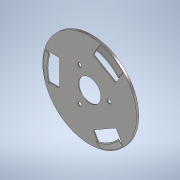
# Autodesk Inventor part: Tarcza_OsłonaB
Saved by Autodesk Inventor 2022 (Build 260153000, 153)
## iProperties
Created: 2021-06-26
Part Number: Tarcza_OsłonaB
Material: Stal, galwanizowana
Document SubType Name: Modeling
Designer: Matik
Density: 7.85 g/cm^3
Appearance: Galwanizowana
Author: Matik
Autodesk Inventor part; units mm, degrees
ref_plane "YZ Plane" through (0, 0, 0) normal (1, 0, 0) x (0, 1, 0)
ref_plane "Płaszczyzna konstrukcyjna1" through (2.025, 0, 2) normal (0, 0, 1) x (-1, 0, 0)
sketch "Szkic1" plane through (2.025, 0, 2) normal (0, 0, 1) x (-1, 0, 0)
  line L0 (22.5, 22.5) -> (22.5, 27.5) projected
  line L1 (22.5, 27.5) -> (27.5, 27.5) projected
  line L2 (27.5, 27.5) -> (27.5, 22.5) projected
  line L3 (27.5, 22.5) -> (22.5, 22.5) projected
  line L4 (-22.5, 27.5) -> (-22.5, 22.5) projected
  line L5 (-22.5, 22.5) -> (-27.5, 22.5) projected
  line L6 (-27.5, 22.5) -> (-27.5, 27.5) projected
  line L7 (-27.5, 27.5) -> (-22.5, 27.5) projected
  line L8 (22.5, -22.5) -> (27.5, -22.5) projected
  line L9 (27.5, -22.5) -> (27.5, -27.5) projected
  line L10 (27.5, -27.5) -> (22.5, -27.5) projected
  line L11 (22.5, -27.5) -> (22.5, -22.5) projected
  line L12 (-27.5, -27.5) -> (-27.5, -22.5) projected
  line L13 (-27.5, -22.5) -> (-22.5, -22.5) projected
  line L14 (-22.5, -22.5) -> (-22.5, -27.5) projected
  line L15 (-22.5, -27.5) -> (-27.5, -27.5) projected
  arc A0 (-56.2827, -21.6239) -> (-57.5723, -24.3244) centre (-55.73, -23.5461) ccw projected
  arc A1 (-57.5723, -24.3244) -> (7.7206, -62.0213) centre (0, 0) ccw projected
  arc A2 (7.7206, -62.0213) -> (9.4144, -59.5542) centre (7.4735, -60.0366) ccw projected
  arc A3 (46.8682, -37.9302) -> (9.4144, -59.5542) centre (31.25, -54.1266) ccw projected
  arc A4 (46.8682, -37.9302) -> (49.8517, -37.6969) centre (48.2565, -36.4906) ccw projected
  arc A5 (49.8517, -37.6969) -> (49.8517, 37.6969) centre (0, 0) ccw projected
  arc A6 (49.8517, 37.6969) -> (46.8682, 37.9302) centre (48.2565, 36.4906) ccw projected
  arc A7 (9.4144, 59.5542) -> (46.8682, 37.9302) centre (31.25, 54.1266) ccw projected
  arc A8 (9.4144, 59.5542) -> (7.7206, 62.0213) centre (7.4735, 60.0366) ccw projected
  arc A9 (7.7206, 62.0213) -> (-57.5723, 24.3244) centre (0, 0) ccw projected
  arc A10 (-57.5723, 24.3244) -> (-56.2827, 21.6239) centre (-55.73, 23.5461) ccw projected
  arc A11 (-56.2827, -21.6239) -> (-56.2827, 21.6239) centre (-62.5, 0) ccw projected
  line L16 (-6.5766, 42.391) -> (-33.4234, 26.891) projected
  arc A12 (-36.1554, 27.6231) -> (-33.4234, 26.891) centre (-34.4234, 28.6231) ccw projected
  line L17 (-36.1554, 27.6231) -> (-42.0186, 37.7784) projected
  arc A13 (-41.9061, 39.9519) -> (-42.0186, 37.7784) centre (-40.2866, 38.7784) ccw projected
  arc A14 (-13.6463, 56.2677) -> (-41.9061, 39.9519) centre (-9.5156, 16.4816) ccw projected
  arc A15 (-11.7077, 55.2784) -> (-13.6463, 56.2677) centre (-13.4398, 54.2784) ccw projected
  line L18 (-11.7077, 55.2784) -> (-5.8446, 45.1231) projected
  arc A16 (-6.5766, 42.391) -> (-5.8446, 45.1231) centre (-7.5766, 44.1231) ccw projected
  line L19 (-33.4234, -26.891) -> (-6.5766, -42.391) projected
  arc A17 (-5.8446, -45.1231) -> (-6.5766, -42.391) centre (-7.5766, -44.1231) ccw projected
  line L20 (-5.8446, -45.1231) -> (-11.7077, -55.2784) projected
  arc A18 (-13.6463, -56.2677) -> (-11.7077, -55.2784) centre (-13.4398, -54.2784) ccw projected
  arc A19 (-41.9061, -39.9519) -> (-13.6463, -56.2677) centre (-9.5156, -16.4816) ccw projected
  arc A20 (-42.0186, -37.7784) -> (-41.9061, -39.9519) centre (-40.2866, -38.7784) ccw projected
  line L21 (-42.0186, -37.7784) -> (-36.1554, -27.6231) projected
  arc A21 (-33.4234, -26.891) -> (-36.1554, -27.6231) centre (-34.4234, -28.6231) ccw projected
  line L22 (40, -15.5) -> (40, 15.5) projected
  arc A22 (42, 17.5) -> (40, 15.5) centre (42, 15.5) ccw projected
  line L23 (42, 17.5) -> (53.7264, 17.5) projected
  arc A23 (55.5524, 16.3158) -> (53.7264, 17.5) centre (53.7264, 15.5) ccw projected
  arc A24 (55.5524, -16.3158) -> (55.5524, 16.3158) centre (19.0313, 0) ccw projected
  arc A25 (53.7264, -17.5) -> (55.5524, -16.3158) centre (53.7264, -15.5) ccw projected
  line L24 (53.7264, -17.5) -> (42, -17.5) projected
  arc A26 (40, -15.5) -> (42, -17.5) centre (42, -15.5) ccw projected
  arc A27 (-21.36, 10) -> (-19.6163, 11.0204) centre (-21.36, 12) ccw projected
  arc A28 (0.2642, 22.4984) -> (-19.6163, 11.0204) centre (0, 0) ccw projected
  arc A29 (0.2642, 22.4984) -> (2.0198, 23.4983) centre (0.2877, 24.4983) ccw projected
  line L25 (2.0198, 23.4983) -> (2.5897, 24.4856) projected
  arc A30 (19.9103, 14.4856) -> (2.5897, 24.4856) centre (11.25, 19.4856) ccw projected
  line L26 (19.9103, 14.4856) -> (19.3403, 13.4983) projected
  arc A31 (19.3403, 13.4983) -> (19.3521, 11.478) centre (21.0723, 12.4983) ccw projected
  arc A32 (19.3521, -11.478) -> (19.3521, 11.478) centre (0, 0) ccw projected
  arc A33 (19.3521, -11.478) -> (19.3403, -13.4983) centre (21.0723, -12.4983) ccw projected
  line L27 (19.3403, -13.4983) -> (19.9103, -14.4856) projected
  arc A34 (2.5897, -24.4856) -> (19.9103, -14.4856) centre (11.25, -19.4856) ccw projected
  line L28 (2.5897, -24.4856) -> (2.0198, -23.4983) projected
  arc A35 (2.0198, -23.4983) -> (0.2642, -22.4984) centre (0.2877, -24.4983) ccw projected
  arc A36 (-19.6163, -11.0204) -> (0.2642, -22.4984) centre (0, 0) ccw projected
  arc A37 (-19.6163, -11.0204) -> (-21.36, -10) centre (-21.36, -12) ccw projected
  line L29 (-21.36, -10) -> (-22.5, -10) projected
  arc A38 (-22.5, 10) -> (-22.5, -10) centre (-22.5, 0) ccw projected
  line L30 (-22.5, 10) -> (-21.36, 10) projected
  circle A39 centre (0, 0) radius 62.5
  circle A40 centre (-26, 0) radius 2.5 projected
  circle A41 centre (13, -22.5167) radius 2.5 projected
  circle A42 centre (13, 22.5167) radius 2.5 projected
  arc A43 (0.2642, 22.4984) -> (-19.6163, 11.0204) centre (0, 0) ccw projected
  arc A44 (-21.36, 10) -> (-19.6163, 11.0204) centre (-21.36, 12) ccw projected
  line L31 (-21.36, 10) -> (-22.5, 10) projected
  arc A45 (-22.5, 10) -> (-22.5, -10) centre (-22.5, 0) ccw projected
  line L32 (-22.5, -10) -> (-21.36, -10) projected
  arc A46 (-19.6163, -11.0204) -> (-21.36, -10) centre (-21.36, -12) ccw projected
  arc A47 (-19.6163, -11.0204) -> (0.2642, -22.4984) centre (0, 0) ccw projected
  arc A48 (2.0198, -23.4983) -> (0.2642, -22.4984) centre (0.2877, -24.4983) ccw projected
  line L33 (2.0198, -23.4983) -> (2.5897, -24.4856) projected
  arc A49 (2.5897, -24.4856) -> (19.9103, -14.4856) centre (11.25, -19.4856) ccw projected
  line L34 (19.9103, -14.4856) -> (19.3403, -13.4983) projected
  arc A50 (19.3521, -11.478) -> (19.3403, -13.4983) centre (21.0723, -12.4983) ccw projected
  arc A51 (19.3521, -11.478) -> (19.3521, 11.478) centre (0, 0) ccw projected
  arc A52 (19.3403, 13.4983) -> (19.3521, 11.478) centre (21.0723, 12.4983) ccw projected
  line L35 (19.3403, 13.4983) -> (19.9103, 14.4856) projected
  arc A53 (19.9103, 14.4856) -> (2.5897, 24.4856) centre (11.25, 19.4856) ccw projected
  line L36 (2.5897, 24.4856) -> (2.0198, 23.4983) projected
  arc A54 (0.2642, 22.4984) -> (2.0198, 23.4983) centre (0.2877, 24.4983) ccw projected
  circle A55 centre (0, 0) radius 15 projected
  point P0 (2.025, 0)
  point P1 (49.8517, -37.6969)
  point P2 (49.8517, 37.6969)
  point P3 (-57.5723, 24.3244)
  point P4 (7.7206, -62.0213)
  constraints: 1 centre point, 1 coincident, 1 concentric
extrude "Wyciągnięcie proste1" add sketch "Szkic1" along normal blind 1 contours L0 L1 L2 L3 | L4 L5 L6 L7 | L8 L9 L10 L11 | L12 L13 L14 L15 | A11 A10 A9 A8 A7 A6 A5 A4 A3 A2 A1 A0 | A0 A39 A10 A11 | A2 A3 A4 A39 | A39 A6 A7 A8 | A27 A28 A29 L25 A30 L26 A31 A32 A33 L27 A34 L28 A35 A36 A37 L29 A38 L30
sketch "Szkic2" plane through (2.025, 0, 2) normal (0, 0, -1) x (-1, 0, 0)
  circle A0 centre (0, 0) radius 61
  circle A1 centre (0, 0) radius 62.5
  point P0 (2.025, 0)
  dimension "d2" = 122
  dimension "d3" = 125
  constraints: 2 centre point, 1 coincident
  measures "d2" diameter of A0
  measures "d3" diameter of A1
extrude "Wyciągnięcie proste2" add sketch "Szkic2" along normal blind 2
ref_plane "Płaszczyzna konstrukcyjna2" through (2.025, 0, 5) normal (0, 0, 1) x (1, 0, 0)
sketch "Szkic5" plane through (2.025, 0, 5) normal (0, 0, 1) x (1, 0, 0)
  arc A0 (-50.7797, 16.8426) -> (-50.7797, -16.8426) centre (0, 0) ccw
  arc A1 (-52.2558, 17.156) -> (-52.2558, -17.156) centre (0, 0) ccw
  line L0 (-42, -17.5) -> (-53.7264, -17.5) projected
  line L1 (-51.2543, -17.5) -> (-51.7808, -17.5)
  line L2 (-53.7264, 17.5) -> (-42, 17.5) projected
  line L3 (-51.2543, 17.5) -> (-51.7808, 17.5)
  arc A2 (-51.2543, -17.5) -> (-50.7797, -16.8426) centre (-51.2543, -17) ccw
  arc A3 (-52.2558, -17.156) -> (-51.7808, -17.5) centre (-51.7808, -17) ccw
  arc A4 (-50.7797, 16.8426) -> (-51.2543, 17.5) centre (-51.2543, 17) ccw
  arc A5 (-51.7808, 17.5) -> (-52.2558, 17.156) centre (-51.7808, 17) ccw
  point P0 (-2.025, 0)
  point P1 (-50.5569, -17.5)
  point P2 (-52.1416, -17.5)
  point P3 (-50.5569, 17.5)
  point P4 (-52.1416, 17.5)
  dimension "d9" = 107
  dimension "d10" = 110
  dimension "d11" = 0.5
  constraints: 16 point on circle, 8 point on line, 8 tangent, 6 centre point, 4 end point, 3 equal radius, 1 coincident
  measures "d9" diameter of A0
  measures "d10" diameter of A1
  measures "d11" radius of A2
sketch "Szkic6" plane through (2.025, 0, 3) normal (0, 0, 1) x (1, 0, 0)
  arc A0 (-59.0635, 17.1393) -> (-59.0635, -17.1393) centre (0, 0) ccw
  arc A1 (-57.5826, 16.8595) -> (-57.5826, -16.8595) centre (0, 0) ccw
  line L0 (-58.0625, -17.5) -> (-58.5833, -17.5)
  line L1 (-58.0625, 17.5) -> (-58.5833, 17.5)
  arc A2 (-58.0625, -17.5) -> (-57.5826, -16.8595) centre (-58.0625, -17) ccw
  arc A3 (-59.0635, -17.1393) -> (-58.5833, -17.5) centre (-58.5833, -17) ccw
  arc A4 (-57.5826, 16.8595) -> (-58.0625, 17.5) centre (-58.0625, 17) ccw
  arc A5 (-58.5833, 17.5) -> (-59.0635, 17.1393) centre (-58.5833, 17) ccw
  point P0 (-2.025, 0)
  point P1 (-57.3912, -17.5)
  point P2 (-58.9576, -17.5)
  point P3 (-57.3912, 17.5)
  point P4 (-58.9576, 17.5)
  dimension "d20" = 123
  dimension "d21" = 120
  dimension "d22" = 0.5
  constraints: 16 point on circle, 8 tangent, 6 centre point, 4 end point, 4 point on line, 3 equal radius, 1 coincident, 1 horizontal, 1 parallel
  measures "d20" diameter of A0
  measures "d21" diameter of A1
  measures "d22" radius of A2
loft "Wyciągnięcie złożone2" add profiles "Szkic6", "Szkic5"
pattern_circular "Szyk kołowy2" count 3 over 360 about axis through (2.025, 0, 2) along (0, 0, 1) of "Wyciągnięcie złożone2"
